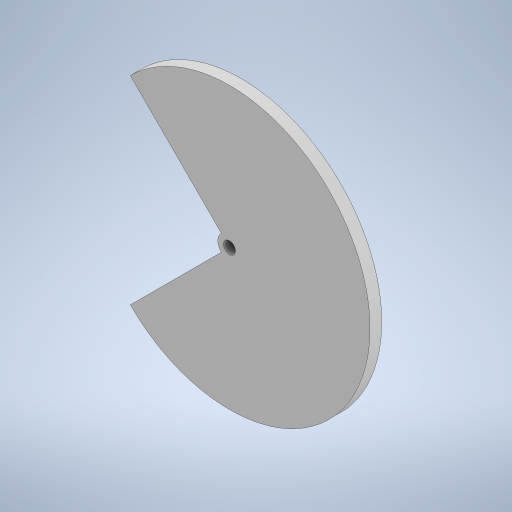
# Autodesk Inventor part: Release1
Saved by Autodesk Inventor 2024 (Build 280153000, 153)
## iProperties
Created: 2023-11-02
Part Number: Release1
Material: Generic
Document SubType Name: Modeling
Designer: flynf
Density: 1 g/cm^3
Appearance: Default
Author: flynf
Autodesk Inventor part; units mm, degrees
ref_plane "YZ Plane" through (0, 0, 0) normal (1, 0, 0) x (0, 1, 0)
ref_plane "XZ Plane" through (0, 0, 0) normal (0, 1, 0) x (-1, 0, 0)
ref_plane "XY Plane" through (0, 0, 0) normal (0, 0, 1) x (1, 0, 0)
sketch "Sketch1" plane through (0, 0, 0) normal (0, 0, 1) x (1, 0, 0)
  circle A0 centre (0, 0) radius 20.32
  circle A1 centre (31.75, 0) radius 38.1
  line L0 (31.75, 0) -> (4.8092, 26.9408)
  line L1 (31.75, 0) -> (4.8092, -26.9408)
  dimension "d0" = 40.64
  dimension "d1" = 90
  dimension "d3" = 0
  dimension "d5" = 31.75
  dimension "d6" = 76.2
  constraints: 4 end point, 2 centre point, 2 point on circle, 1 coincident
  measures "d0" diameter of A0
  measures "d1" angle of L0 L1
  measures "d3" vertical distance of point (0, 0) L0.start
  measures "d5" distance of point (0, 0) L0.start
  measures "d6" diameter of A1
extrude "Extrusion1" add sketch "Sketch1" along normal blind 3.175 contours A1 L1 L0
sketch "Sketch2" plane through (0, 0, 3.175) normal (0, 0, 1) x (1, 0, 0)
  line L0 (31.75, 0) -> (4.8092, -26.9408) projected
  circle A0 centre (31.75, 0) radius 1.5875
  circle A1 centre (31.75, 0) radius 3.175
  point P0 (0, 0)
  dimension "d10" = 3.175
  dimension "d11" = 6.35
  constraints: 2 centre point, 1 coincident
  measures "d10" diameter of A0
  measures "d11" diameter of A1
extrude "Extrusion2" add sketch "Sketch2" against normal blind 3.175
sketch "Sketch3" plane through (0, 0, 3.175) normal (0, 0, 1) x (1, 0, 0)
  line L0 (31.75, 0) -> (30.6275, -1.1225) projected
  circle A0 centre (31.75, 0) radius 1.5875
  point P0 (0, 0)
  constraints: 1 centre point
extrude "Extrusion3" cut sketch "Sketch3" against normal blind 3.175
body "Solid1"
